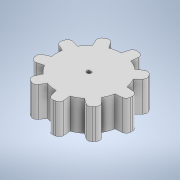
# Autodesk Inventor part: KOŁO
Saved by Autodesk Inventor 2022 (Build 260153000, 153)
## iProperties
Created: 2022-04-03
Part Number: KOŁO
Material: Ogólny
Document SubType Name: Modeling
Designer: jolow
Density: 1 g/cm^3
Appearance: Domyślna
Author: jolow
Autodesk Inventor part; units mm, degrees
ref_plane "YZ Plane" through (0, 0, 0) normal (1, 0, 0) x (0, 1, 0)
ref_plane "XZ Plane" through (0, 0, 0) normal (0, 1, 0) x (-1, 0, 0)
ref_plane "XY Plane" through (0, 0, 0) normal (0, 0, 1) x (1, 0, 0)
sketch "Szkic1" plane through (0, 0, 0) normal (0, 1, 0) x (-1, 0, 0)
  circle A0 centre (0, 0) radius 22.5
  dimension "d0" = 45
  constraints: 1 centre point, 1 coincident
  measures "d0" diameter of A0
extrude "Wyciągnięcie proste1" add sketch "Szkic1" along normal blind 21
sketch "Szkic2" plane through (0, 21, 0) normal (0, 1, 0) x (1, 0, 0)
  circle A0 centre (0, 0) radius 22.5 projected
  line L0 (22.1151, -4.144) -> (29.5, -3.5)
  line L1 (29.5, -3.5) -> (29.5, 3.5)
  line L2 (29.5, 3.5) -> (22.1151, 4.144)
  line L3 (22.1151, -4.144) -> (22.1151, 4.144)
  dimension "d3" = 7
  dimension "d4" = 7
  constraints: 8 end point, 2 point on circle, 1 equal length, 1 parallel, 1 vertical
  measures "d3" distance edge to line of A0 L1
  measures "d4" distance of L0.end L1.end
extrude "Wyciągnięcie proste2" add sketch "Szkic2" against normal blind 21 contours A0 L2 L1 L0
fillet "Zaokrąglenie1" radius 3 2 edges at (29.5, 10.5, -3.5) (29.5, 10.5, 3.5)
pattern_circular "Szyk kołowy2" count 9 over 360 about axis through (0, 0, 0) along (0, 1, 0) of "Wyciągnięcie proste2", "Zaokrąglenie1"
sketch "Szkic3" plane through (0, 0, 0) normal (0, -1, 0) x (1, 0, 0)
  point P0 (0, 0)
sketch "Szkic4" plane through (0, 21, 0) normal (0, 1, 0) x (1, 0, 0)
  circle A0 centre (0, 0) radius 1.5
  line L0 (-1.118, 1) -> (1.118, 1)
  circle A1 centre (0, 0) radius 2
  dimension "d14" = 3
  dimension "d15" = 2.5
  dimension "d16" = 0
  dimension "d17" = 0
  constraints: 2 centre point, 2 end point, 2 point on circle
  measures "d14" diameter of A0
  measures "d16" distance of A1.centre A0.centre
  measures "d17" distance of A1.centre A0.centre
extrude "Wyciągnięcie proste3" cut sketch "Szkic4" against normal through all contours A0 L0 picked at (0.0594, 0.1702)
